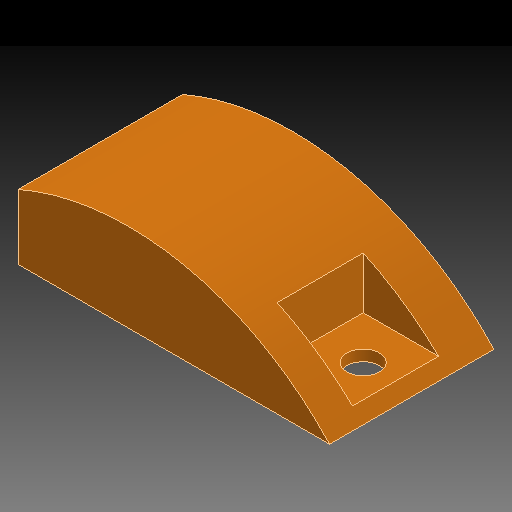
# Autodesk Inventor part: KB33-046-002-006 - Заглушка
Saved by Autodesk Inventor 2020 (Build 240168000, 168)
## iProperties
Created: 2021-07-29
Part Number: KB33-046-002-006 - Заглушка
Material: Типовые
Document SubType Name: Modeling
Designer: Петров Иван
Mass: 2.49199 g
Surface Area: 13.8961 cm^2
Volume: 2.49199 cm^3
Density: 1 g/cm^3
Appearance: Оранжевый
Author: Петров Иван
Autodesk Inventor part; units mm, degrees
ref_plane "YZ Plane" through (0, 0, 0) normal (1, 0, 0) x (0, 1, 0)
ref_plane "XZ Plane" through (0, 0, 0) normal (0, 1, 0) x (-1, 0, 0)
sketch "Эскиз1" plane through (0, 0, 0) normal (0, 0, 1) x (1, 0, 0)
  arc A0 (28.4298, -5.9319) -> (0, 0) centre (10.0583, -22.8873) ccw
  line L0 (0, -5.9315) -> (0, 0)
  line L1 (23.9975, -5.9315) -> (0, -5.9315)
  line L2 (23.9975, -5.9315) -> (23.998, -5.9315)
  line L3 (23.998, -5.9319) -> (23.998, -5.9315)
  line L4 (23.998, -5.9319) -> (28.4298, -5.9319)
  point P0 (0, 0)
  point P1 (-10.0583, 22.8873)
  constraints: 10 end point, 2 point on circle, 1 centre point, 1 horizontal
extrude "Выдавливание1" add sketch "Эскиз1" along normal blind 15
ref_plane "РабПлоскость1" through (10.0583, 2.1127, 0) normal (0, -1, 0) x (1, 0, 0)
sketch "Эскиз2" plane through (10.0583, 2.1127, 0) normal (0, -1, 0) x (1, 0, 0)
  circle A0 centre (14.4417, 8) radius 1.5 projected
  line L0 (18.3715, 0) -> (18.3715, 15) projected
  line L1 (10.5118, 11.93) -> (18.3715, 11.93)
  line L2 (18.3715, 11.93) -> (18.3715, 4.07)
  line L3 (18.3715, 4.07) -> (10.5118, 4.07)
  line L4 (10.5118, 4.07) -> (10.5118, 11.93)
  line L5 (10.5118, 11.93) -> (18.3715, 4.07) construction
  line L6 (18.3715, 11.93) -> (10.5118, 4.07) construction
  point P0 (-10.0583, 0)
  dimension "d2" = 7.86
  constraints: 12 end point, 2 midpoint, 2 parallel, 1 horizontal, 1 perpendicular, 1 point on line
  measures "d2" distance of L1.end L2.end
extrude "Выдавливание2" cut sketch "Эскиз2" along normal blind 10.2942 contours A0
sketch "Эскиз3" plane through (10.0583, 2.1127, 0) normal (0, -1, 0) x (1, 0, 0)
  circle A0 centre (14.4417, 8) radius 1.5
  line L0 (18.3715, 0) -> (18.3715, 15)
  line L1 (10.5118, 11.93) -> (18.3715, 11.93)
  line L2 (18.3715, 11.93) -> (18.3715, 4.07)
  line L3 (18.3715, 4.07) -> (10.5118, 4.07)
  line L4 (10.5118, 4.07) -> (10.5118, 11.93)
  line L5 (10.5118, 11.93) -> (18.3715, 4.07) construction
  line L6 (18.3715, 11.93) -> (10.5118, 4.07) construction
  point P0 (-10.0583, 0)
  point P1 (-10.0583, 0)
  dimension "d5" = 7.86
  constraints: 14 end point, 2 midpoint, 2 parallel, 1 centre point, 1 horizontal, 1 perpendicular, 1 point on line
  measures "d5" distance of L1.end L2.end
extrude "Выдавливание3" cut sketch "Эскиз3" along normal blind 7.0442
